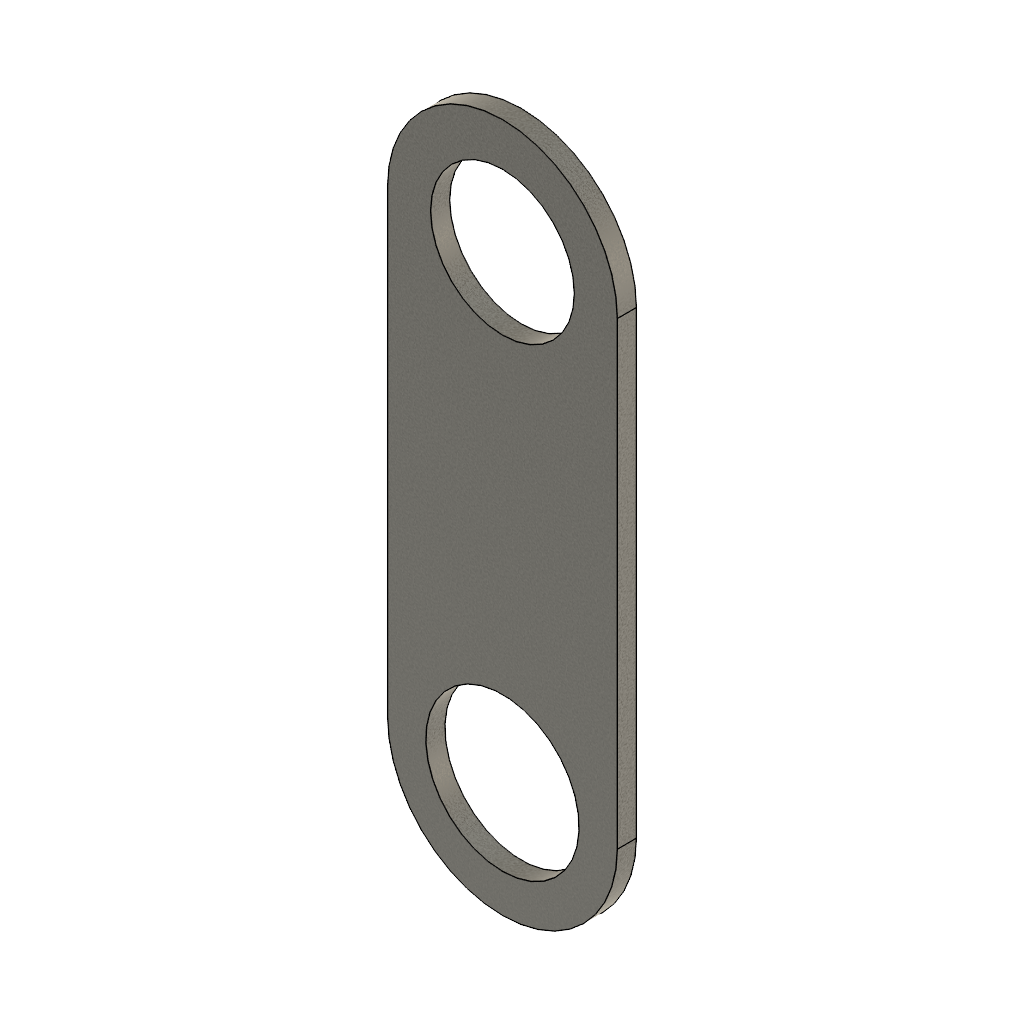
A6-Link (Autodesk Fusion 360 design; units mm, degrees)
part number: 2026-09-28-08-44-29-713
Autodesk Fusion 360 part; units mm, degrees
sketch "Sketch1" plane through (0, 0, 0) normal (0, 1, 0) x (1, 0, 0)
  arc A0 (38.1, -12.7) -> (0, -12.7) centre (19.05, -12.7) ccw
  line L0 (0, -12.7) -> (0, -88.9)
  line L1 (38.1, -12.7) -> (38.1, -88.9)
  arc A1 (0, -88.9) -> (38.1, -88.9) centre (19.05, -88.9) ccw
  dimension "d9" = 76.2
  dimension "d11" = 38.1
  constraint tangent A0 L0
  constraint vertical L0
  constraint tangent A0 L1
  constraint vertical L1
  constraint tangent L1 A1
  constraint tangent L0 A1
  measures "d9" distance of A0.centre A1.centre
  measures "d11" distance of L0 L1
extrude "Extrude1" add sketch "Sketch1" along normal blind 3.175
hole "Hole1" at (19.05, 0, 88.9) direction (0, 1, 0) diameter 23.8125 end through all
hole "Hole2" at (19.05, 0, 12.7) direction (0, 1, 0) diameter 25.4 end through all
equation "L = 3 in"
equation "P = 500 lbforce"
equation "stress = 9000 psi"
equation "d_A = 0.9375 in"
equation "d_1 = 1 in"
equation "t = ceil(( P / ( d_A * stress ) ) / 0.125 in) * 0.125 in"
equation "d9 = L"
equation "d11 = w"
equation "w = 1.5 in"
equation "d13 = t"
equation "d15 = d_A"
equation "d17 = d_1"
